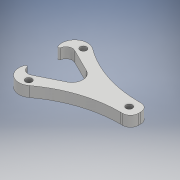
# Autodesk Inventor part: legFrame_short
Saved by Autodesk Inventor 2017 (Build 210142000, 142)
## iProperties
Created: 2016-08-27
Part Number: legFrame_short
Material: Generic
Document SubType Name: Modeling
Designer: Nic
Density: 1 g/cm^3
Appearance: Default
Author: Nic
Autodesk Inventor part; units mm, degrees
ref_plane "YZ Plane" through (0, 0, 0) normal (1, 0, 0) x (0, 1, 0)
ref_plane "XZ Plane" through (0, 0, 0) normal (0, 1, 0) x (-1, 0, 0)
ref_plane "XY Plane" through (0, 0, 0) normal (0, 0, 1) x (1, 0, 0)
sketch "Sketch1" plane through (0, 0, 0) normal (0, 0, 1) x (1, 0, 0)
  circle A0 centre (0, 0) radius 1.25
  circle A1 centre (-28.1025, 10.5) radius 1.25
  circle A2 centre (-28.1025, -10.5) radius 1.25
  line L0 (0, 0) -> (-28.1025, 0) construction
  line L1 (-28.1025, 10.5) -> (0, 0) construction
  line L2 (-28.1025, 0) -> (-28.1025, 10.5) construction
  circle A3 centre (0, 0) radius 2.5 construction
  circle A4 centre (-28.1025, 10.5) radius 2.5 construction
  circle A5 centre (-28.1025, -10.5) radius 2.5 construction
  line L3 (0, 0) -> (0, 7) construction
  line L4 (0, 3.5) -> (1, 3.5)
  arc A6 (-26.277, 12.2081) -> (0, 3.5) centre (0, 47.5) ccw
  line L5 (0, -3.5) -> (1, -3.5)
  arc A7 (-20.1367, -3.7476) -> (-20.1367, 3.7476) centre (-22, 0) ccw
  arc A8 (-26.277, 12.2081) -> (-33.7448, 6.3389) centre (-29.2155, 8.2614) ccw
  line L6 (-20.1367, 3.7476) -> (-29.2155, 8.2614)
  arc A9 (-29.2155, 8.2614) -> (-32.7919, 6.449) centre (-30.3285, 6.0228) ccw
  arc A10 (-33.7448, 6.3389) -> (-32.7919, 6.449) centre (-33.2846, 6.5343) ccw
  arc A11 (0, -3.5) -> (-26.277, -12.2081) centre (0, -47.5) ccw
  arc A12 (-33.7448, -6.3389) -> (-26.277, -12.2081) centre (-29.2155, -8.2614) ccw
  line L7 (-20.1367, -3.7476) -> (-29.2155, -8.2614)
  arc A13 (-32.7919, -6.449) -> (-29.2155, -8.2614) centre (-30.3285, -6.0228) ccw
  arc A14 (-32.7919, -6.449) -> (-33.7448, -6.3389) centre (-33.2846, -6.5343) ccw
  line L8 (4, 0.5) -> (4, -0.5)
  arc A15 (4, 0.5) -> (1, 3.5) centre (1, 0.5) ccw
  arc A16 (1, -3.5) -> (4, -0.5) centre (1, -0.5) ccw
  dimension "d0" = 2.5
  dimension "d1" = 10.5
  dimension "d2" = 30
  dimension "d3" = 5
  dimension "d22" = 3.5
  dimension "d32" = 0.5
  dimension "d36" = 22
  dimension "d37" = 2.5
  dimension "d38" = 0.5
  dimension "d47" = 44
  dimension "d48" = 4
  dimension "d49" = 3
  constraints: 26 point on circle, 18 end point, 17 centre point, 13 tangent, 9 symmetric about line, 6 coincident, 5 equal radius, 3 horizontal, 2 vertical, 1 perpendicular, 1 point on line, 1 vertical alignment, 4 other
  measures "d0" diameter of A0
  measures "d1" distance of L0.end L1.start
  measures "d2" distance of L1.start L0.start
  measures "d3" diameter of A3
  measures "d22" distance from line of point (0, 0) L4
  measures "d32" radius of A10
  measures "d36" distance of point (0, 0) A7.centre
  measures "d37" radius of A9
  measures "d38" radius of A14
  measures "d47" radius of A6
  measures "d48" distance from line of point (0, 0) L8
  measures "d49" radius of A15
extrude "Extrusion1" add sketch "Sketch1" along normal blind 4
body "Solid1"
